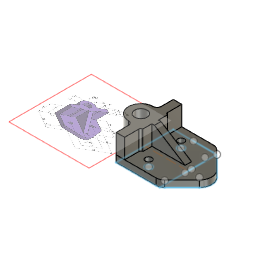
A3 v3 (Autodesk Fusion 360 design; units mm, degrees)
Autodesk Fusion 360 part; units mm, degrees
sketch "base" plane through (0, 0, 0) normal (0, 0, 1) x (1, 0, 0)
  line L0 (75, -35) -> (136.6142, -35)
  line L1 (142, -35) -> (142, 53)
  line L2 (136.6142, 53) -> (75, 53)
  line L3 (75, 53) -> (75, -35)
  line L4 (142, 9) -> (142, 14)
  line L5 (142, 9) -> (142, 4)
  line L6 (136.6142, 53) -> (106, 53)
  line L7 (142, 9) -> (142, 34)
  circle A0 centre (106, 34) radius 5
  line L8 (142, 9) -> (75, 9) construction
  circle A1 centre (106, -16) radius 5
  line L9 (145.8078, -31.1912) -> (172.5588, -4.4333)
  line L10 (172.5588, 22.4333) -> (145.8078, 49.1912)
  arc A2 (172.5588, -4.4333) -> (172.5588, 22.4333) centre (159.122, 9) ccw
  arc A3 (136.6142, -35) -> (145.8078, -31.1912) centre (136.6142, -22) ccw
  arc A4 (145.8078, 49.1912) -> (136.6142, 53) centre (136.6142, 40) ccw
  dimension "d1" = 67
  dimension "d2" = 88
  dimension "d3" = 5
  dimension "d4" = 5
  dimension "d5" = 36
  dimension "d6" = 25
  dimension "d7" = 10
  dimension "d8" = 19
  dimension "d9" = 13
  dimension "d10" = 13
  constraint horizontal L0
  constraint vertical L1
  constraint horizontal L2
  constraint vertical L3
  constraint midpoint L1 L4.start
  constraint perpendicular L0 L4
  constraint parallel L1 L5
  constraint perpendicular L1 L6
  constraint coincident L1 L7.end
  constraint midpoint L3 L8.end
  constraint symmetric A0 L8 A1
  constraint tangent L9 A2
  constraint tangent L10 A2
  constraint coincident L1.start L9
  constraint coincident L1.start L0
  constraint tangent L9 A3
  constraint tangent L0 A3
  constraint coincident L1.end L10
  constraint coincident L1.end L6
  constraint tangent L10 A4
  constraint tangent L6 A4
  measures "d1" distance of L0.start L1.start
  measures "d2" distance of L0.start L2.end
  measures "d3" distance of L4.start L4.end
  measures "d4" distance of L4.start L5.end
  measures "d5" distance of L1.end L6.end
  measures "d6" distance of L4.start L7.end
  measures "d7" diameter of A0
  measures "d8" radius of A2
  measures "d9" radius of A3
  measures "d10" radius of A4
extrude "Extrude1" add sketch "base" along normal blind 10
sketch "top" plane through (0, 0, 10) normal (0, 0, 1) x (-1, 0, 0)
  circle A0 centre (-106, 16) radius 5
  circle A1 centre (-106, -34) radius 5
  arc A2 (-145.8078, -49.1912) -> (-136.6142, -53) centre (-136.6142, -40) ccw
  line L0 (-136.6142, -53) -> (-75, -53)
  line L1 (-75, -53) -> (-75, 35)
  line L2 (-75, 35) -> (-136.6142, 35)
  arc A3 (-136.6142, 35) -> (-145.8078, 31.1912) centre (-136.6142, 22) ccw
  line L3 (-145.8078, 31.1912) -> (-172.5588, 4.4333)
  arc A4 (-172.5588, 4.4333) -> (-172.5588, -22.4333) centre (-159.122, -9) ccw
  line L4 (-172.5588, -22.4333) -> (-145.8078, -49.1912)
  line L5 (-75, -53) -> (-88, -53)
  circle A5 centre (-69, -9) radius 9.5
  line L6 (-142, -14) -> (-95, -14)
  line L7 (-142, -14) -> (-142, -4)
  line L8 (-142, -4) -> (-95, -4)
  line L9 (-95, -4) -> (-95, -14)
  line L10 (-91, -9) -> (-91, -28)
  line L11 (-91, -28) -> (-91, -9)
  line L12 (-91, -9) -> (-91, 10)
  line L13 (-91, -28) -> (-91, -28)
  line L14 (-88, -31) -> (-88, -53)
  line L15 (-91, 10) -> (-91, 10)
  line L16 (-88, 13) -> (-88, 35)
  arc A6 (-88, -31) -> (-91, -28) centre (-91, -31) ccw
  arc A7 (-91, 10) -> (-88, 13) centre (-91, 13) ccw
  line L17 (-95, -14) -> (-91, -14)
  line L18 (-91, -4) -> (-95, -4)
  line L19 (-75, -53) -> (-75, -34)
  line L20 (-88, 35) -> (-75, 35)
  line L21 (-75, 35) -> (-75, 16)
  line L22 (-69, -28) -> (-69, -28)
  arc A8 (-69, -28) -> (-75, -34) centre (-69, -34) ccw
  line L23 (-69, 10) -> (-69, 10)
  arc A9 (-75, 16) -> (-69, 10) centre (-69, 16) ccw
  arc A10 (-69, -28) -> (-69, 10) centre (-69, -9) ccw
  dimension "d13" = 19
  dimension "d14" = 3
  dimension "d15" = 3
  dimension "d16" = 6
  dimension "d17" = 6
  constraint coincident L0.end L1.start
  constraint coincident L0 L5.end
  constraint perpendicular L1 L5
  constraint parallel L0 L6
  constraint perpendicular L6 L7
  constraint perpendicular L7 L8
  constraint perpendicular L6 L9
  constraint parallel L1 L10
  constraint parallel L10 L11
  constraint parallel L11 L12
  constraint perpendicular L0 L14
  constraint coincident L2 L16.end
  constraint perpendicular L2 L16
  constraint tangent L14 A6
  constraint tangent L16 A7
  constraint coincident L11 L17.end
  constraint perpendicular L11 L17
  constraint coincident L12 L18.start
  constraint perpendicular L9 L18
  constraint perpendicular L0 L19
  constraint coincident L1.end L2.start
  constraint parallel L1 L21
  constraint tangent L19 A8
  constraint tangent L21 A9
  constraint tangent A8 A10
  measures "d13" diameter of A5
  measures "d14" radius of A6
  measures "d15" radius of A7
  measures "d16" radius of A8
  measures "d17" radius of A9
extrude "Extrude2" add sketch "top" against normal blind 10 contours L1 A5 A8 A9 A10
extrude "Extrude3" add sketch "top" along normal blind 30 contours L6 L7 L8 L9
sketch "ramp" plane through (0, 4, 0) normal (0, -1, 0) x (1, 0, 0)
  line L0 (95, 10) -> (142, 10)
  line L1 (142, 10) -> (142, 40)
  line L2 (142, 40) -> (95, 40)
  line L3 (95, 40) -> (95, 10)
  line L4 (95, 40) -> (142, 10)
  line L5 (142, 10) -> (142, 40)
  line L6 (95, 40) -> (142, 40)
  constraint coincident L2.end L3.start
  constraint coincident L0.end L1.start
  constraint coincident L1.end L2.start
extrude "Extrude4" cut sketch "ramp" against normal blind 10 contours L1 L2 L4 L5 L6
extrude "Extrude5" add sketch "top" along normal blind 30 contours L9 L10 L11 L12 L17 L18
extrude "Extrude6" add sketch "top" along normal blind 30 contours L0 L1 L2 L5 A5 L10 L11 L12 L14 L16 A6 A7 L19 L20 L21
extrude "Extrude7" add sketch "top" along normal blind 30 contours L1 A5 A8 A9 A10
extrude "Extrude8" cut 1 faces at (75.8602, 7.6409, 10) along direction (0, 0, -1) blind 10
